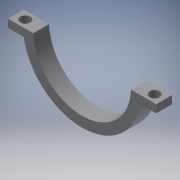
# Autodesk Inventor part: MOTOR MOUNT REAL TOP E3O MOTOR
Saved by Autodesk Inventor 2019 (Build 230136000, 136)
## iProperties
Created: 2018-01-16
Part Number: MOTOR MOUNT REAL TOP E3O MOTOR
Material: Generic
Document SubType Name: Modeling
Designer: Administrator
Density: 1 g/cm^3
Appearance: Default
Author: Administrator
Autodesk Inventor part; units mm, degrees
ref_plane "YZ Plane" through (0, 0, 0) normal (1, 0, 0) x (0, 1, 0)
ref_plane "XZ Plane" through (0, 0, 0) normal (0, 1, 0) x (-1, 0, 0)
ref_plane "XY Plane" through (0, 0, 0) normal (0, 0, 1) x (1, 0, 0)
sketch "Sketch1" plane through (0, 0, 0) normal (0, 0, 1) x (1, 0, 0)
  arc A0 (-39.344, -1.4316) -> (39.344, -1.4316) centre (0, 0) ccw
  line L0 (-39.344, -1.4316) -> (-39.3671, -1.4316)
  line L1 (-39.344, -1.4316) -> (-52.044, -1.4316)
  line L2 (39.344, -1.4316) -> (52.044, -1.4316)
  arc A1 (-46.964, -22.4724) -> (46.964, -22.4724) centre (0, 0) ccw
  line L3 (-52.044, -1.4316) -> (-59.664, -1.4316)
  line L4 (52.044, -1.4316) -> (59.664, -1.4316)
  line L5 (39.344, -1.4316) -> (46.964, -1.4316)
  line L6 (46.964, -1.4316) -> (46.964, -22.4724)
  line L7 (-39.344, -1.4316) -> (-45.694, -1.4316)
  line L8 (-39.344, -1.4316) -> (-46.964, -1.4316)
  line L9 (-46.964, -1.4316) -> (-46.964, -22.4724)
  line L10 (-46.964, -7.7816) -> (-59.664, -7.7816)
  line L11 (-59.664, -7.7816) -> (-59.664, -1.4316)
  line L12 (46.964, -7.7816) -> (59.664, -7.7816)
  line L13 (59.664, -7.7816) -> (59.664, -1.4316)
  line L14 (46.964, -42.5386) -> (30.0181, -42.5386)
  line L15 (46.964, -22.4724) -> (46.964, -42.5386)
  line L16 (46.964, -42.5386) -> (-46.964, -42.5386)
  line L17 (-46.964, -42.5386) -> (-46.964, -22.4724)
  line L18 (-46.964, -42.5386) -> (46.964, -42.5386)
  line L19 (46.964, -42.5386) -> (46.964, -52.2316)
  line L20 (46.964, -52.2316) -> (-46.964, -52.2316)
  line L21 (-46.964, -52.2316) -> (-46.964, -42.5386)
  line L22 (-46.964, -22.4724) -> (-32.3263, -22.4724)
  line L23 (32.3263, -22.4724) -> (46.964, -22.4724)
  dimension "d0" = 78.74
  dimension "d1" = 12.7
  dimension "d2" = 12.7
  dimension "d4" = 7.62
  dimension "d5" = 7.62
  dimension "d6" = 7.62
  dimension "d7" = 7.62
  dimension "d8" = 6.35
  dimension "d9" = 6.35
  dimension "d20" = 50.8
  constraints: 48 end point, 8 horizontal, 7 point on circle, 6 point on line, 5 parallel, 5 perpendicular, 2 centre point, 2 vertical, 1 coincident, 1 concentric, 1 midpoint
  measures "d0" diameter of A0
  measures "d1" distance of L2.start L2.end
  measures "d2" distance of L0.start L1.end
  measures "d4" distance of L1.end L11.end
  measures "d5" distance of L2.end L13.end
  measures "d6" distance of L2.start L5.end
  measures "d7" distance of L0.start L8.end
  measures "d8" distance of L10.end L11.end
  measures "d9" distance of L12.end L13.end
  measures "d20" distance between parallel lines of L5 L20
extrude "Extrusion1" add sketch "Sketch1" along normal blind 12.7
sketch "Sketch2" plane through (-59.664, -1.4316, 0) normal (0, 1, 0) x (1, 0, 0)
  line L0 (20.32, 0) -> (0, 0) projected
  line L1 (0, 0) -> (20.32, 0)
  circle A0 centre (7.62, -6.35) radius 4.064
  circle A1 centre (111.7079, -6.35) radius 4.064
  line L2 (99.0079, 0) -> (99.0079, -12.7) projected
  line L3 (20.32, 0) -> (20.32, -12.7) projected
  point P0 (59.664, 0)
  dimension "d14" = 12.7
  dimension "d15" = 12.7
  dimension "d16" = 8.128
  dimension "d17" = 8.128
  constraints: 2 centre point, 2 end point, 1 horizontal
  measures "d14" distance from line of L2 A1.centre
  measures "d15" distance from line of L3 A0.centre
  measures "d16" diameter of A0
  measures "d17" diameter of A1
extrude "Extrusion2" cut sketch "Sketch2" against normal blind 25.4
body "Solid1"
